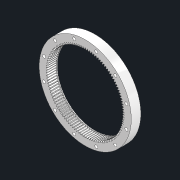
# Autodesk Inventor part: unit-ring_gear
Saved by Autodesk Inventor 2021 (Build 250183000, 183)
## iProperties
Created: 2021-07-12
Part Number: unit-ring_gear
Material: ABS プラスチック
Document SubType Name: Modeling
Designer: yuta0
Density: 1.06 g/cm^3
Appearance: 滑らか - 白
Mass: 40.8022 g
Surface Area: 244.347 cm^2
Volume: 38.4926 cm^3
Author: yuta0
Autodesk Inventor part; units mm, degrees
ref_plane "YZ Plane" through (0, 0, 0) normal (1, 0, 0) x (0, 1, 0)
ref_plane "XZ Plane" through (0, 0, 0) normal (0, 1, 0) x (-1, 0, 0)
ref_plane "XY Plane" through (0, 0, 0) normal (0, 0, 1) x (1, 0, 0)
sketch "スケッチ1" plane through (0, 0, 0) normal (0, 0, 1) x (1, 0, 0)
  arc A0 (3.605, -57.0442) -> (4.2313, -54.7448) centre (-9.8704, -52.1391) ccw
  arc A1 (2.8046, -57.0892) -> (3.605, -57.0442) centre (0, 0) ccw
  arc A2 (1.9248, -54.8743) -> (2.8046, -57.0892) centre (15.6461, -50.7061) ccw
  arc A3 (1.155, -54.8959) -> (1.9248, -54.8743) centre (0, 0) ccw
  arc A4 (0.4008, -57.1566) -> (1.155, -54.8959) centre (-12.7783, -51.5036) ccw
  arc A5 (-0.4008, -57.1566) -> (0.4008, -57.1566) centre (0, 0) ccw
  arc A6 (-1.155, -54.8959) -> (-0.4008, -57.1566) centre (12.7783, -51.5036) ccw
  arc A7 (-1.9248, -54.8743) -> (-1.155, -54.8959) centre (0, 0) ccw
  arc A8 (-2.8046, -57.0892) -> (-1.9248, -54.8743) centre (-15.6461, -50.7061) ccw
  arc A9 (-3.605, -57.0442) -> (-2.8046, -57.0892) centre (0, 0) ccw
  arc A10 (-4.2313, -54.7448) -> (-3.605, -57.0442) centre (9.8704, -52.1391) ccw
  arc A11 (-4.9986, -54.68) -> (-4.2313, -54.7448) centre (0, 0) ccw
  arc A12 (-6.0012, -56.8421) -> (-4.9986, -54.68) centre (-18.4646, -49.7491) ccw
  arc A13 (-6.7978, -56.7524) -> (-6.0012, -56.8421) centre (0, 0) ccw
  arc A14 (-7.2942, -54.4214) -> (-6.7978, -56.7524) centre (6.9314, -52.6105) ccw
  arc A15 (-8.0567, -54.3137) -> (-7.2942, -54.4214) centre (0, 0) ccw
  arc A16 (-9.1789, -56.4162) -> (-8.0567, -54.3137) centre (-21.225, -48.6355) ccw
  arc A17 (-9.9692, -56.2819) -> (-9.1789, -56.4162) centre (0, 0) ccw
  arc A18 (-10.3341, -53.9268) -> (-9.9692, -56.2819) centre (3.9706, -52.9164) ccw
  arc A19 (-11.0894, -53.7765) -> (-10.3341, -53.9268) centre (0, 0) ccw
  arc A20 (-12.3278, -55.8128) -> (-11.0894, -53.7765) centre (-23.9186, -47.3689) ccw
  arc A21 (-13.1093, -55.6344) -> (-12.3278, -55.8128) centre (0, 0) ccw
  arc A22 (-13.3416, -53.2625) -> (-13.1093, -55.6344) centre (0.9973, -53.0558) ccw
  arc A23 (-14.0872, -53.0702) -> (-13.3416, -53.2625) centre (0, 0) ccw
  arc A24 (-15.4378, -55.0337) -> (-14.0872, -53.0702) centre (-26.537, -45.9533) ccw
  arc A25 (-16.2081, -54.8118) -> (-15.4378, -55.0337) centre (0, 0) ccw
  arc A26 (-16.307, -52.4306) -> (-16.2081, -54.8118) centre (-1.9791, -53.0282) ccw
  arc A27 (-17.0407, -52.1968) -> (-16.307, -52.4306) centre (0, 0) ccw
  arc A28 (-18.4993, -54.0816) -> (-17.0407, -52.1968) centre (-29.0718, -44.393) ccw
  arc A29 (-19.256, -53.8168) -> (-18.4993, -54.0816) centre (0, 0) ccw
  arc A30 (-19.2212, -51.4338) -> (-19.256, -53.8168) centre (-4.9493, -52.8339) ccw
  arc A31 (-19.9406, -51.1592) -> (-19.2212, -51.4338) centre (0, 0) ccw
  arc A32 (-21.5026, -52.9592) -> (-19.9406, -51.1592) centre (-31.5152, -42.6931) ccw
  arc A33 (-22.2432, -52.6524) -> (-21.5026, -52.9592) centre (0, 0) ccw
  arc A34 (-22.0749, -50.2752) -> (-22.2432, -52.6524) centre (-7.904, -52.4732) ccw
  arc A35 (-22.7778, -49.9606) -> (-22.0749, -50.2752) centre (0, 0) ccw
  arc A36 (-24.4382, -51.6702) -> (-22.7778, -49.9606) centre (-33.8595, -40.8589) ccw
  arc A37 (-25.1605, -51.3224) -> (-24.4382, -51.6702) centre (0, 0) ccw
  arc A38 (-24.8591, -48.9583) -> (-25.1605, -51.3224) centre (-10.8337, -51.9475) ccw
  arc A39 (-25.5433, -48.6049) -> (-24.8591, -48.9583) centre (0, 0) ccw
  arc A40 (-27.2969, -50.2187) -> (-25.5433, -48.6049) centre (-36.0972, -38.8961) ccw
  arc A41 (-27.9985, -49.8309) -> (-27.2969, -50.2187) centre (0, 0) ccw
  arc A42 (-27.5651, -47.4874) -> (-27.9985, -49.8309) centre (-13.7294, -51.2583) ccw
  arc A43 (-28.2284, -47.0962) -> (-27.5651, -47.4874) centre (0, 0) ccw
  arc A44 (-30.0698, -48.6091) -> (-28.2284, -47.0962) centre (-38.2213, -36.8109) ccw
  arc A45 (-30.7485, -48.1826) -> (-30.0698, -48.6091) centre (0, 0) ccw
  arc A46 (-30.1844, -45.8671) -> (-30.7485, -48.1826) centre (-16.5819, -50.4079) ccw
  arc A47 (-30.8247, -45.4393) -> (-30.1844, -45.8671) centre (0, 0) ccw
  arc A48 (-32.748, -46.8466) -> (-30.8247, -45.4393) centre (-40.2252, -34.6099) ccw
  arc A49 (-33.4018, -46.3828) -> (-32.748, -46.8466) centre (0, 0) ccw
  arc A50 (-32.7087, -44.1025) -> (-33.4018, -46.3828) centre (-19.3822, -49.3988) ccw
  arc A51 (-33.324, -43.6395) -> (-32.7087, -44.1025) centre (0, 0) ccw
  arc A52 (-35.3232, -44.9368) -> (-33.324, -43.6395) centre (-42.1025, -32.3) ccw
  arc A53 (-35.9499, -44.4369) -> (-35.3232, -44.9368) centre (0, 0) ccw
  arc A54 (-35.1301, -42.1992) -> (-35.9499, -44.4369) centre (-22.1215, -48.2343) ccw
  arc A55 (-35.7184, -41.7023) -> (-35.1301, -42.1992) centre (0, 0) ccw
  arc A56 (-37.7873, -42.8855) -> (-35.7184, -41.7023) centre (-43.8473, -29.8885) ccw
  arc A57 (-38.385, -42.3513) -> (-37.7873, -42.8855) centre (0, 0) ccw
  arc A58 (-37.4409, -40.163) -> (-38.385, -42.3513) centre (-24.7912, -46.9181) ccw
  arc A59 (-38.0005, -39.634) -> (-37.4409, -40.163) centre (0, 0) ccw
  arc A60 (-40.1324, -40.6993) -> (-38.0005, -39.634) centre (-45.4542, -27.3829) ccw
  arc A61 (-40.6993, -40.1324) -> (-40.1324, -40.6993) centre (0, 0) ccw
  arc A62 (-39.634, -38.0005) -> (-40.6993, -40.1324) centre (-27.3829, -45.4542) ccw
  arc A63 (-40.163, -37.4409) -> (-39.634, -38.0005) centre (0, 0) ccw
  arc A64 (-42.3513, -38.385) -> (-40.163, -37.4409) centre (-46.9181, -24.7912) ccw
  arc A65 (-42.8855, -37.7873) -> (-42.3513, -38.385) centre (0, 0) ccw
  arc A66 (-41.7023, -35.7184) -> (-42.8855, -37.7873) centre (-29.8885, -43.8473) ccw
  arc A67 (-42.1992, -35.1301) -> (-41.7023, -35.7184) centre (0, 0) ccw
  arc A68 (-44.4369, -35.9499) -> (-42.1992, -35.1301) centre (-48.2343, -22.1215) ccw
  arc A69 (-44.9368, -35.3232) -> (-44.4369, -35.9499) centre (0, 0) ccw
  arc A70 (-43.6395, -33.324) -> (-44.9368, -35.3232) centre (-32.3, -42.1025) ccw
  arc A71 (-44.1025, -32.7087) -> (-43.6395, -33.324) centre (0, 0) ccw
  arc A72 (-46.3828, -33.4018) -> (-44.1025, -32.7087) centre (-49.3988, -19.3822) ccw
  arc A73 (-46.8466, -32.748) -> (-46.3828, -33.4018) centre (0, 0) ccw
  arc A74 (-45.4393, -30.8247) -> (-46.8466, -32.748) centre (-34.6099, -40.2252) ccw
  arc A75 (-45.8671, -30.1844) -> (-45.4393, -30.8247) centre (0, 0) ccw
  arc A76 (-48.1826, -30.7485) -> (-45.8671, -30.1844) centre (-50.4079, -16.5819) ccw
  arc A77 (-48.6091, -30.0698) -> (-48.1826, -30.7485) centre (0, 0) ccw
  arc A78 (-47.0962, -28.2284) -> (-48.6091, -30.0698) centre (-36.8109, -38.2213) ccw
  arc A79 (-47.4874, -27.5651) -> (-47.0962, -28.2284) centre (0, 0) ccw
  arc A80 (-49.8309, -27.9985) -> (-47.4874, -27.5651) centre (-51.2583, -13.7294) ccw
  arc A81 (-50.2187, -27.2969) -> (-49.8309, -27.9985) centre (0, 0) ccw
  arc A82 (-48.6049, -25.5433) -> (-50.2187, -27.2969) centre (-38.8961, -36.0972) ccw
  arc A83 (-48.9583, -24.8591) -> (-48.6049, -25.5433) centre (0, 0) ccw
  arc A84 (-51.3224, -25.1605) -> (-48.9583, -24.8591) centre (-51.9475, -10.8337) ccw
  arc A85 (-51.6702, -24.4382) -> (-51.3224, -25.1605) centre (0, 0) ccw
  arc A86 (-49.9606, -22.7778) -> (-51.6702, -24.4382) centre (-40.8589, -33.8595) ccw
  arc A87 (-50.2752, -22.0749) -> (-49.9606, -22.7778) centre (0, 0) ccw
  arc A88 (-52.6524, -22.2432) -> (-50.2752, -22.0749) centre (-52.4732, -7.904) ccw
  arc A89 (-52.9592, -21.5026) -> (-52.6524, -22.2432) centre (0, 0) ccw
  arc A90 (-51.1592, -19.9406) -> (-52.9592, -21.5026) centre (-42.6931, -31.5152) ccw
  arc A91 (-51.4338, -19.2212) -> (-51.1592, -19.9406) centre (0, 0) ccw
  arc A92 (-53.8168, -19.256) -> (-51.4338, -19.2212) centre (-52.8339, -4.9493) ccw
  arc A93 (-54.0816, -18.4993) -> (-53.8168, -19.256) centre (0, 0) ccw
  arc A94 (-52.1968, -17.0407) -> (-54.0816, -18.4993) centre (-44.393, -29.0718) ccw
  arc A95 (-52.4306, -16.307) -> (-52.1968, -17.0407) centre (0, 0) ccw
  arc A96 (-54.8118, -16.2081) -> (-52.4306, -16.307) centre (-53.0282, -1.9791) ccw
  arc A97 (-55.0337, -15.4378) -> (-54.8118, -16.2081) centre (0, 0) ccw
  arc A98 (-53.0702, -14.0872) -> (-55.0337, -15.4378) centre (-45.9533, -26.537) ccw
  arc A99 (-53.2625, -13.3416) -> (-53.0702, -14.0872) centre (0, 0) ccw
  arc A100 (-55.6344, -13.1093) -> (-53.2625, -13.3416) centre (-53.0558, 0.9973) ccw
  arc A101 (-55.8128, -12.3278) -> (-55.6344, -13.1093) centre (0, 0) ccw
  arc A102 (-53.7765, -11.0894) -> (-55.8128, -12.3278) centre (-47.3689, -23.9186) ccw
  arc A103 (-53.9268, -10.3341) -> (-53.7765, -11.0894) centre (0, 0) ccw
  arc A104 (-56.2819, -9.9692) -> (-53.9268, -10.3341) centre (-52.9164, 3.9706) ccw
  arc A105 (-56.4162, -9.1789) -> (-56.2819, -9.9692) centre (0, 0) ccw
  arc A106 (-54.3137, -8.0567) -> (-56.4162, -9.1789) centre (-48.6355, -21.225) ccw
  arc A107 (-54.4214, -7.2942) -> (-54.3137, -8.0567) centre (0, 0) ccw
  arc A108 (-56.7524, -6.7978) -> (-54.4214, -7.2942) centre (-52.6105, 6.9314) ccw
  arc A109 (-56.8421, -6.0012) -> (-56.7524, -6.7978) centre (0, 0) ccw
  arc A110 (-54.68, -4.9986) -> (-56.8421, -6.0012) centre (-49.7491, -18.4646) ccw
  arc A111 (-54.7448, -4.2313) -> (-54.68, -4.9986) centre (0, 0) ccw
  arc A112 (-57.0442, -3.605) -> (-54.7448, -4.2313) centre (-52.1391, 9.8704) ccw
  arc A113 (-57.0892, -2.8046) -> (-57.0442, -3.605) centre (0, 0) ccw
  arc A114 (-54.8743, -1.9248) -> (-57.0892, -2.8046) centre (-50.7061, -15.6461) ccw
  arc A115 (-54.8959, -1.155) -> (-54.8743, -1.9248) centre (0, 0) ccw
  arc A116 (-57.1566, -0.4008) -> (-54.8959, -1.155) centre (-51.5036, 12.7783) ccw
  arc A117 (-57.1566, 0.4008) -> (-57.1566, -0.4008) centre (0, 0) ccw
  arc A118 (-54.8959, 1.155) -> (-57.1566, 0.4008) centre (-51.5036, -12.7783) ccw
  arc A119 (-54.8743, 1.9248) -> (-54.8959, 1.155) centre (0, 0) ccw
  arc A120 (-57.0892, 2.8046) -> (-54.8743, 1.9248) centre (-50.7061, 15.6461) ccw
  arc A121 (-57.0442, 3.605) -> (-57.0892, 2.8046) centre (0, 0) ccw
  arc A122 (-54.7448, 4.2313) -> (-57.0442, 3.605) centre (-52.1391, -9.8704) ccw
  arc A123 (-54.68, 4.9986) -> (-54.7448, 4.2313) centre (0, 0) ccw
  arc A124 (-56.8421, 6.0012) -> (-54.68, 4.9986) centre (-49.7491, 18.4646) ccw
  arc A125 (-56.7524, 6.7978) -> (-56.8421, 6.0012) centre (0, 0) ccw
  arc A126 (-54.4214, 7.2942) -> (-56.7524, 6.7978) centre (-52.6105, -6.9314) ccw
  arc A127 (-54.3137, 8.0567) -> (-54.4214, 7.2942) centre (0, 0) ccw
  arc A128 (-56.4162, 9.1789) -> (-54.3137, 8.0567) centre (-48.6355, 21.225) ccw
  arc A129 (-56.2819, 9.9692) -> (-56.4162, 9.1789) centre (0, 0) ccw
  arc A130 (-53.9268, 10.3341) -> (-56.2819, 9.9692) centre (-52.9164, -3.9706) ccw
  arc A131 (-53.7765, 11.0894) -> (-53.9268, 10.3341) centre (0, 0) ccw
  arc A132 (-55.8128, 12.3278) -> (-53.7765, 11.0894) centre (-47.3689, 23.9186) ccw
  arc A133 (-55.6344, 13.1093) -> (-55.8128, 12.3278) centre (0, 0) ccw
  arc A134 (-53.2625, 13.3416) -> (-55.6344, 13.1093) centre (-53.0558, -0.9973) ccw
  arc A135 (-53.0702, 14.0872) -> (-53.2625, 13.3416) centre (0, 0) ccw
  arc A136 (-55.0337, 15.4378) -> (-53.0702, 14.0872) centre (-45.9533, 26.537) ccw
  arc A137 (-54.8118, 16.2081) -> (-55.0337, 15.4378) centre (0, 0) ccw
  arc A138 (-52.4306, 16.307) -> (-54.8118, 16.2081) centre (-53.0282, 1.9791) ccw
  arc A139 (-52.1968, 17.0407) -> (-52.4306, 16.307) centre (0, 0) ccw
  arc A140 (-54.0816, 18.4993) -> (-52.1968, 17.0407) centre (-44.393, 29.0718) ccw
  arc A141 (-53.8168, 19.256) -> (-54.0816, 18.4993) centre (0, 0) ccw
  arc A142 (-51.4338, 19.2212) -> (-53.8168, 19.256) centre (-52.8339, 4.9493) ccw
  arc A143 (-51.1592, 19.9406) -> (-51.4338, 19.2212) centre (0, 0) ccw
  arc A144 (-52.9592, 21.5026) -> (-51.1592, 19.9406) centre (-42.6931, 31.5152) ccw
  arc A145 (-52.6524, 22.2432) -> (-52.9592, 21.5026) centre (0, 0) ccw
  arc A146 (-50.2752, 22.0749) -> (-52.6524, 22.2432) centre (-52.4732, 7.904) ccw
  arc A147 (-49.9606, 22.7778) -> (-50.2752, 22.0749) centre (0, 0) ccw
  arc A148 (-51.6702, 24.4382) -> (-49.9606, 22.7778) centre (-40.8589, 33.8595) ccw
  arc A149 (-51.3224, 25.1605) -> (-51.6702, 24.4382) centre (0, 0) ccw
  arc A150 (-48.9583, 24.8591) -> (-51.3224, 25.1605) centre (-51.9475, 10.8337) ccw
  arc A151 (-48.6049, 25.5433) -> (-48.9583, 24.8591) centre (0, 0) ccw
  arc A152 (-50.2187, 27.2969) -> (-48.6049, 25.5433) centre (-38.8961, 36.0972) ccw
  arc A153 (-49.8309, 27.9985) -> (-50.2187, 27.2969) centre (0, 0) ccw
  arc A154 (-47.4874, 27.5651) -> (-49.8309, 27.9985) centre (-51.2583, 13.7294) ccw
  arc A155 (-47.0962, 28.2284) -> (-47.4874, 27.5651) centre (0, 0) ccw
  arc A156 (-48.6091, 30.0698) -> (-47.0962, 28.2284) centre (-36.8109, 38.2213) ccw
  arc A157 (-48.1826, 30.7485) -> (-48.6091, 30.0698) centre (0, 0) ccw
  arc A158 (-45.8671, 30.1844) -> (-48.1826, 30.7485) centre (-50.4079, 16.5819) ccw
  arc A159 (-45.4393, 30.8247) -> (-45.8671, 30.1844) centre (0, 0) ccw
  arc A160 (-46.8466, 32.748) -> (-45.4393, 30.8247) centre (-34.6099, 40.2252) ccw
  arc A161 (-46.3828, 33.4018) -> (-46.8466, 32.748) centre (0, 0) ccw
  arc A162 (-44.1025, 32.7087) -> (-46.3828, 33.4018) centre (-49.3988, 19.3822) ccw
  arc A163 (-43.6395, 33.324) -> (-44.1025, 32.7087) centre (0, 0) ccw
  arc A164 (-44.9368, 35.3232) -> (-43.6395, 33.324) centre (-32.3, 42.1025) ccw
  arc A165 (-44.4369, 35.9499) -> (-44.9368, 35.3232) centre (0, 0) ccw
  arc A166 (-42.1992, 35.1301) -> (-44.4369, 35.9499) centre (-48.2343, 22.1215) ccw
  arc A167 (-41.7023, 35.7184) -> (-42.1992, 35.1301) centre (0, 0) ccw
  arc A168 (-42.8855, 37.7873) -> (-41.7023, 35.7184) centre (-29.8885, 43.8473) ccw
  arc A169 (-42.3513, 38.385) -> (-42.8855, 37.7873) centre (0, 0) ccw
  arc A170 (-40.163, 37.4409) -> (-42.3513, 38.385) centre (-46.9181, 24.7912) ccw
  arc A171 (-39.634, 38.0005) -> (-40.163, 37.4409) centre (0, 0) ccw
  arc A172 (-40.6993, 40.1324) -> (-39.634, 38.0005) centre (-27.3829, 45.4542) ccw
  arc A173 (-40.1324, 40.6993) -> (-40.6993, 40.1324) centre (0, 0) ccw
  arc A174 (-38.0005, 39.634) -> (-40.1324, 40.6993) centre (-45.4542, 27.3829) ccw
  arc A175 (-37.4409, 40.163) -> (-38.0005, 39.634) centre (0, 0) ccw
  arc A176 (-38.385, 42.3513) -> (-37.4409, 40.163) centre (-24.7912, 46.9181) ccw
  arc A177 (-37.7873, 42.8855) -> (-38.385, 42.3513) centre (0, 0) ccw
  arc A178 (-35.7184, 41.7023) -> (-37.7873, 42.8855) centre (-43.8473, 29.8885) ccw
  arc A179 (-35.1301, 42.1992) -> (-35.7184, 41.7023) centre (0, 0) ccw
  arc A180 (-35.9499, 44.4369) -> (-35.1301, 42.1992) centre (-22.1215, 48.2343) ccw
  arc A181 (-35.3232, 44.9368) -> (-35.9499, 44.4369) centre (0, 0) ccw
  arc A182 (-33.324, 43.6395) -> (-35.3232, 44.9368) centre (-42.1025, 32.3) ccw
  arc A183 (-32.7087, 44.1025) -> (-33.324, 43.6395) centre (0, 0) ccw
  arc A184 (-33.4018, 46.3828) -> (-32.7087, 44.1025) centre (-19.3822, 49.3988) ccw
  arc A185 (-32.748, 46.8466) -> (-33.4018, 46.3828) centre (0, 0) ccw
  arc A186 (-30.8247, 45.4393) -> (-32.748, 46.8466) centre (-40.2252, 34.6099) ccw
  arc A187 (-30.1844, 45.8671) -> (-30.8247, 45.4393) centre (0, 0) ccw
  arc A188 (-30.7485, 48.1826) -> (-30.1844, 45.8671) centre (-16.5819, 50.4079) ccw
  arc A189 (-30.0698, 48.6091) -> (-30.7485, 48.1826) centre (0, 0) ccw
  arc A190 (-28.2284, 47.0962) -> (-30.0698, 48.6091) centre (-38.2213, 36.8109) ccw
  arc A191 (-27.5651, 47.4874) -> (-28.2284, 47.0962) centre (0, 0) ccw
  arc A192 (-27.9985, 49.8309) -> (-27.5651, 47.4874) centre (-13.7294, 51.2583) ccw
  arc A193 (-27.2969, 50.2187) -> (-27.9985, 49.8309) centre (0, 0) ccw
  arc A194 (-25.5433, 48.6049) -> (-27.2969, 50.2187) centre (-36.0972, 38.8961) ccw
  arc A195 (-24.8591, 48.9583) -> (-25.5433, 48.6049) centre (0, 0) ccw
  arc A196 (-25.1605, 51.3224) -> (-24.8591, 48.9583) centre (-10.8337, 51.9475) ccw
  arc A197 (-24.4382, 51.6702) -> (-25.1605, 51.3224) centre (0, 0) ccw
  arc A198 (-22.7778, 49.9606) -> (-24.4382, 51.6702) centre (-33.8595, 40.8589) ccw
  arc A199 (-22.0749, 50.2752) -> (-22.7778, 49.9606) centre (0, 0) ccw
  arc A200 (-22.2432, 52.6524) -> (-22.0749, 50.2752) centre (-7.904, 52.4732) ccw
  arc A201 (-21.5026, 52.9592) -> (-22.2432, 52.6524) centre (0, 0) ccw
  arc A202 (-19.9406, 51.1592) -> (-21.5026, 52.9592) centre (-31.5152, 42.6931) ccw
  arc A203 (-19.2212, 51.4338) -> (-19.9406, 51.1592) centre (0, 0) ccw
  arc A204 (-19.256, 53.8168) -> (-19.2212, 51.4338) centre (-4.9493, 52.8339) ccw
  arc A205 (-18.4993, 54.0816) -> (-19.256, 53.8168) centre (0, 0) ccw
  arc A206 (-17.0407, 52.1968) -> (-18.4993, 54.0816) centre (-29.0718, 44.393) ccw
  arc A207 (-16.307, 52.4306) -> (-17.0407, 52.1968) centre (0, 0) ccw
  arc A208 (-16.2081, 54.8118) -> (-16.307, 52.4306) centre (-1.9791, 53.0282) ccw
  arc A209 (-15.4378, 55.0337) -> (-16.2081, 54.8118) centre (0, 0) ccw
  arc A210 (-14.0872, 53.0702) -> (-15.4378, 55.0337) centre (-26.537, 45.9533) ccw
  arc A211 (-13.3416, 53.2625) -> (-14.0872, 53.0702) centre (0, 0) ccw
  arc A212 (-13.1093, 55.6344) -> (-13.3416, 53.2625) centre (0.9973, 53.0558) ccw
  arc A213 (-12.3278, 55.8128) -> (-13.1093, 55.6344) centre (0, 0) ccw
  arc A214 (-11.0894, 53.7765) -> (-12.3278, 55.8128) centre (-23.9186, 47.3689) ccw
  arc A215 (-10.3341, 53.9268) -> (-11.0894, 53.7765) centre (0, 0) ccw
  arc A216 (-9.9692, 56.2819) -> (-10.3341, 53.9268) centre (3.9706, 52.9164) ccw
  arc A217 (-9.1789, 56.4162) -> (-9.9692, 56.2819) centre (0, 0) ccw
  arc A218 (-8.0567, 54.3137) -> (-9.1789, 56.4162) centre (-21.225, 48.6355) ccw
  arc A219 (-7.2942, 54.4214) -> (-8.0567, 54.3137) centre (0, 0) ccw
  arc A220 (-6.7978, 56.7524) -> (-7.2942, 54.4214) centre (6.9314, 52.6105) ccw
  arc A221 (-6.0012, 56.8421) -> (-6.7978, 56.7524) centre (0, 0) ccw
  arc A222 (-4.9986, 54.68) -> (-6.0012, 56.8421) centre (-18.4646, 49.7491) ccw
  arc A223 (-4.2313, 54.7448) -> (-4.9986, 54.68) centre (0, 0) ccw
  arc A224 (-3.605, 57.0442) -> (-4.2313, 54.7448) centre (9.8704, 52.1391) ccw
  arc A225 (-2.8046, 57.0892) -> (-3.605, 57.0442) centre (0, 0) ccw
  arc A226 (-1.9248, 54.8743) -> (-2.8046, 57.0892) centre (-15.6461, 50.7061) ccw
  arc A227 (-1.155, 54.8959) -> (-1.9248, 54.8743) centre (0, 0) ccw
  arc A228 (-0.4008, 57.1566) -> (-1.155, 54.8959) centre (12.7783, 51.5036) ccw
  arc A229 (0.4008, 57.1566) -> (-0.4008, 57.1566) centre (0, 0) ccw
  arc A230 (1.155, 54.8959) -> (0.4008, 57.1566) centre (-12.7783, 51.5036) ccw
  arc A231 (1.9248, 54.8743) -> (1.155, 54.8959) centre (0, 0) ccw
  arc A232 (2.8046, 57.0892) -> (1.9248, 54.8743) centre (15.6461, 50.7061) ccw
  arc A233 (3.605, 57.0442) -> (2.8046, 57.0892) centre (0, 0) ccw
  arc A234 (4.2313, 54.7448) -> (3.605, 57.0442) centre (-9.8704, 52.1391) ccw
  arc A235 (4.9986, 54.68) -> (4.2313, 54.7448) centre (0, 0) ccw
  arc A236 (6.0012, 56.8421) -> (4.9986, 54.68) centre (18.4646, 49.7491) ccw
  arc A237 (6.7978, 56.7524) -> (6.0012, 56.8421) centre (0, 0) ccw
  arc A238 (7.2942, 54.4214) -> (6.7978, 56.7524) centre (-6.9314, 52.6105) ccw
  arc A239 (8.0567, 54.3137) -> (7.2942, 54.4214) centre (0, 0) ccw
  arc A240 (9.1789, 56.4162) -> (8.0567, 54.3137) centre (21.225, 48.6355) ccw
  arc A241 (9.9692, 56.2819) -> (9.1789, 56.4162) centre (0, 0) ccw
  arc A242 (10.3341, 53.9268) -> (9.9692, 56.2819) centre (-3.9706, 52.9164) ccw
  arc A243 (11.0894, 53.7765) -> (10.3341, 53.9268) centre (0, 0) ccw
  arc A244 (12.3278, 55.8128) -> (11.0894, 53.7765) centre (23.9186, 47.3689) ccw
  arc A245 (13.1093, 55.6344) -> (12.3278, 55.8128) centre (0, 0) ccw
  arc A246 (13.3416, 53.2625) -> (13.1093, 55.6344) centre (-0.9973, 53.0558) ccw
  arc A247 (14.0872, 53.0702) -> (13.3416, 53.2625) centre (0, 0) ccw
  arc A248 (15.4378, 55.0337) -> (14.0872, 53.0702) centre (26.537, 45.9533) ccw
  arc A249 (16.2081, 54.8118) -> (15.4378, 55.0337) centre (0, 0) ccw
  arc A250 (16.307, 52.4306) -> (16.2081, 54.8118) centre (1.9791, 53.0282) ccw
  arc A251 (17.0407, 52.1968) -> (16.307, 52.4306) centre (0, 0) ccw
  arc A252 (18.4993, 54.0816) -> (17.0407, 52.1968) centre (29.0718, 44.393) ccw
  arc A253 (19.256, 53.8168) -> (18.4993, 54.0816) centre (0, 0) ccw
  arc A254 (19.2212, 51.4338) -> (19.256, 53.8168) centre (4.9493, 52.8339) ccw
  arc A255 (19.9406, 51.1592) -> (19.2212, 51.4338) centre (0, 0) ccw
  arc A256 (21.5026, 52.9592) -> (19.9406, 51.1592) centre (31.5152, 42.6931) ccw
  arc A257 (22.2432, 52.6524) -> (21.5026, 52.9592) centre (0, 0) ccw
  arc A258 (22.0749, 50.2752) -> (22.2432, 52.6524) centre (7.904, 52.4732) ccw
  arc A259 (22.7778, 49.9606) -> (22.0749, 50.2752) centre (0, 0) ccw
  arc A260 (24.4382, 51.6702) -> (22.7778, 49.9606) centre (33.8595, 40.8589) ccw
  arc A261 (25.1605, 51.3224) -> (24.4382, 51.6702) centre (0, 0) ccw
  arc A262 (24.8591, 48.9583) -> (25.1605, 51.3224) centre (10.8337, 51.9475) ccw
  arc A263 (25.5433, 48.6049) -> (24.8591, 48.9583) centre (0, 0) ccw
  arc A264 (27.2969, 50.2187) -> (25.5433, 48.6049) centre (36.0972, 38.8961) ccw
  arc A265 (27.9985, 49.8309) -> (27.2969, 50.2187) centre (0, 0) ccw
  arc A266 (27.5651, 47.4874) -> (27.9985, 49.8309) centre (13.7294, 51.2583) ccw
  arc A267 (28.2284, 47.0962) -> (27.5651, 47.4874) centre (0, 0) ccw
  arc A268 (30.0698, 48.6091) -> (28.2284, 47.0962) centre (38.2213, 36.8109) ccw
  arc A269 (30.7485, 48.1826) -> (30.0698, 48.6091) centre (0, 0) ccw
  arc A270 (30.1844, 45.8671) -> (30.7485, 48.1826) centre (16.5819, 50.4079) ccw
  arc A271 (30.8247, 45.4393) -> (30.1844, 45.8671) centre (0, 0) ccw
  arc A272 (32.748, 46.8466) -> (30.8247, 45.4393) centre (40.2252, 34.6099) ccw
  arc A273 (33.4018, 46.3828) -> (32.748, 46.8466) centre (0, 0) ccw
  arc A274 (32.7087, 44.1025) -> (33.4018, 46.3828) centre (19.3822, 49.3988) ccw
  arc A275 (33.324, 43.6395) -> (32.7087, 44.1025) centre (0, 0) ccw
  arc A276 (35.3232, 44.9368) -> (33.324, 43.6395) centre (42.1025, 32.3) ccw
  arc A277 (35.9499, 44.4369) -> (35.3232, 44.9368) centre (0, 0) ccw
  arc A278 (35.1301, 42.1992) -> (35.9499, 44.4369) centre (22.1215, 48.2343) ccw
  arc A279 (35.7184, 41.7023) -> (35.1301, 42.1992) centre (0, 0) ccw
  arc A280 (37.7873, 42.8855) -> (35.7184, 41.7023) centre (43.8473, 29.8885) ccw
  arc A281 (38.385, 42.3513) -> (37.7873, 42.8855) centre (0, 0) ccw
  arc A282 (37.4409, 40.163) -> (38.385, 42.3513) centre (24.7912, 46.9181) ccw
  arc A283 (38.0005, 39.634) -> (37.4409, 40.163) centre (0, 0) ccw
  arc A284 (40.1324, 40.6993) -> (38.0005, 39.634) centre (45.4542, 27.3829) ccw
  arc A285 (40.6993, 40.1324) -> (40.1324, 40.6993) centre (0, 0) ccw
  arc A286 (39.634, 38.0005) -> (40.6993, 40.1324) centre (27.3829, 45.4542) ccw
  arc A287 (40.163, 37.4409) -> (39.634, 38.0005) centre (0, 0) ccw
  arc A288 (42.3513, 38.385) -> (40.163, 37.4409) centre (46.9181, 24.7912) ccw
  arc A289 (42.8855, 37.7873) -> (42.3513, 38.385) centre (0, 0) ccw
  arc A290 (41.7023, 35.7184) -> (42.8855, 37.7873) centre (29.8885, 43.8473) ccw
  arc A291 (42.1992, 35.1301) -> (41.7023, 35.7184) centre (0, 0) ccw
  arc A292 (44.4369, 35.9499) -> (42.1992, 35.1301) centre (48.2343, 22.1215) ccw
  arc A293 (44.9368, 35.3232) -> (44.4369, 35.9499) centre (0, 0) ccw
  arc A294 (43.6395, 33.324) -> (44.9368, 35.3232) centre (32.3, 42.1025) ccw
  arc A295 (44.1025, 32.7087) -> (43.6395, 33.324) centre (0, 0) ccw
  arc A296 (46.3828, 33.4018) -> (44.1025, 32.7087) centre (49.3988, 19.3822) ccw
  arc A297 (46.8466, 32.748) -> (46.3828, 33.4018) centre (0, 0) ccw
  arc A298 (45.4393, 30.8247) -> (46.8466, 32.748) centre (34.6099, 40.2252) ccw
  arc A299 (45.8671, 30.1844) -> (45.4393, 30.8247) centre (0, 0) ccw
  arc A300 (48.1826, 30.7485) -> (45.8671, 30.1844) centre (50.4079, 16.5819) ccw
  arc A301 (48.6091, 30.0698) -> (48.1826, 30.7485) centre (0, 0) ccw
  arc A302 (47.0962, 28.2284) -> (48.6091, 30.0698) centre (36.8109, 38.2213) ccw
  arc A303 (47.4874, 27.5651) -> (47.0962, 28.2284) centre (0, 0) ccw
  arc A304 (49.8309, 27.9985) -> (47.4874, 27.5651) centre (51.2583, 13.7294) ccw
  arc A305 (50.2187, 27.2969) -> (49.8309, 27.9985) centre (0, 0) ccw
  arc A306 (48.6049, 25.5433) -> (50.2187, 27.2969) centre (38.8961, 36.0972) ccw
  arc A307 (48.9583, 24.8591) -> (48.6049, 25.5433) centre (0, 0) ccw
  arc A308 (51.3224, 25.1605) -> (48.9583, 24.8591) centre (51.9475, 10.8337) ccw
  arc A309 (51.6702, 24.4382) -> (51.3224, 25.1605) centre (0, 0) ccw
  arc A310 (49.9606, 22.7778) -> (51.6702, 24.4382) centre (40.8589, 33.8595) ccw
  arc A311 (50.2752, 22.0749) -> (49.9606, 22.7778) centre (0, 0) ccw
  arc A312 (52.6524, 22.2432) -> (50.2752, 22.0749) centre (52.4732, 7.904) ccw
  arc A313 (52.9592, 21.5026) -> (52.6524, 22.2432) centre (0, 0) ccw
  arc A314 (51.1592, 19.9406) -> (52.9592, 21.5026) centre (42.6931, 31.5152) ccw
  arc A315 (51.4338, 19.2212) -> (51.1592, 19.9406) centre (0, 0) ccw
  arc A316 (53.8168, 19.256) -> (51.4338, 19.2212) centre (52.8339, 4.9493) ccw
  arc A317 (54.0816, 18.4993) -> (53.8168, 19.256) centre (0, 0) ccw
  arc A318 (52.1968, 17.0407) -> (54.0816, 18.4993) centre (44.393, 29.0718) ccw
  arc A319 (52.4306, 16.307) -> (52.1968, 17.0407) centre (0, 0) ccw
  arc A320 (54.8118, 16.2081) -> (52.4306, 16.307) centre (53.0282, 1.9791) ccw
  arc A321 (55.0337, 15.4378) -> (54.8118, 16.2081) centre (0, 0) ccw
  arc A322 (53.0702, 14.0872) -> (55.0337, 15.4378) centre (45.9533, 26.537) ccw
  arc A323 (53.2625, 13.3416) -> (53.0702, 14.0872) centre (0, 0) ccw
  arc A324 (55.6344, 13.1093) -> (53.2625, 13.3416) centre (53.0558, -0.9973) ccw
  arc A325 (55.8128, 12.3278) -> (55.6344, 13.1093) centre (0, 0) ccw
  arc A326 (53.7765, 11.0894) -> (55.8128, 12.3278) centre (47.3689, 23.9186) ccw
  arc A327 (53.9268, 10.3341) -> (53.7765, 11.0894) centre (0, 0) ccw
  arc A328 (56.2819, 9.9692) -> (53.9268, 10.3341) centre (52.9164, -3.9706) ccw
  arc A329 (56.4162, 9.1789) -> (56.2819, 9.9692) centre (0, 0) ccw
  arc A330 (54.3137, 8.0567) -> (56.4162, 9.1789) centre (48.6355, 21.225) ccw
  arc A331 (54.4214, 7.2942) -> (54.3137, 8.0567) centre (0, 0) ccw
  arc A332 (56.7524, 6.7978) -> (54.4214, 7.2942) centre (52.6105, -6.9314) ccw
  arc A333 (56.8421, 6.0012) -> (56.7524, 6.7978) centre (0, 0) ccw
  arc A334 (54.68, 4.9986) -> (56.8421, 6.0012) centre (49.7491, 18.4646) ccw
  arc A335 (54.7448, 4.2313) -> (54.68, 4.9986) centre (0, 0) ccw
  arc A336 (57.0442, 3.605) -> (54.7448, 4.2313) centre (52.1391, -9.8704) ccw
  arc A337 (57.0892, 2.8046) -> (57.0442, 3.605) centre (0, 0) ccw
  arc A338 (54.8743, 1.9248) -> (57.0892, 2.8046) centre (50.7061, 15.6461) ccw
  arc A339 (54.8959, 1.155) -> (54.8743, 1.9248) centre (0, 0) ccw
  arc A340 (57.1566, 0.4008) -> (54.8959, 1.155) centre (51.5036, -12.7783) ccw
  arc A341 (57.1566, -0.4008) -> (57.1566, 0.4008) centre (0, 0) ccw
  arc A342 (54.8959, -1.155) -> (57.1566, -0.4008) centre (51.5036, 12.7783) ccw
  arc A343 (54.8743, -1.9248) -> (54.8959, -1.155) centre (0, 0) ccw
  arc A344 (57.0892, -2.8046) -> (54.8743, -1.9248) centre (50.7061, -15.6461) ccw
  arc A345 (57.0442, -3.605) -> (57.0892, -2.8046) centre (0, 0) ccw
  arc A346 (54.7448, -4.2313) -> (57.0442, -3.605) centre (52.1391, 9.8704) ccw
  arc A347 (54.68, -4.9986) -> (54.7448, -4.2313) centre (0, 0) ccw
  arc A348 (56.8421, -6.0012) -> (54.68, -4.9986) centre (49.7491, -18.4646) ccw
  arc A349 (56.7524, -6.7978) -> (56.8421, -6.0012) centre (0, 0) ccw
  arc A350 (54.4214, -7.2942) -> (56.7524, -6.7978) centre (52.6105, 6.9314) ccw
  arc A351 (54.3137, -8.0567) -> (54.4214, -7.2942) centre (0, 0) ccw
  arc A352 (56.4162, -9.1789) -> (54.3137, -8.0567) centre (48.6355, -21.225) ccw
  arc A353 (56.2819, -9.9692) -> (56.4162, -9.1789) centre (0, 0) ccw
  arc A354 (53.9268, -10.3341) -> (56.2819, -9.9692) centre (52.9164, 3.9706) ccw
  arc A355 (53.7765, -11.0894) -> (53.9268, -10.3341) centre (0, 0) ccw
  arc A356 (55.8128, -12.3278) -> (53.7765, -11.0894) centre (47.3689, -23.9186) ccw
  arc A357 (55.6344, -13.1093) -> (55.8128, -12.3278) centre (0, 0) ccw
  arc A358 (53.2625, -13.3416) -> (55.6344, -13.1093) centre (53.0558, 0.9973) ccw
  arc A359 (53.0702, -14.0872) -> (53.2625, -13.3416) centre (0, 0) ccw
  arc A360 (55.0337, -15.4378) -> (53.0702, -14.0872) centre (45.9533, -26.537) ccw
  arc A361 (54.8118, -16.2081) -> (55.0337, -15.4378) centre (0, 0) ccw
  arc A362 (52.4306, -16.307) -> (54.8118, -16.2081) centre (53.0282, -1.9791) ccw
  arc A363 (52.1968, -17.0407) -> (52.4306, -16.307) centre (0, 0) ccw
  arc A364 (54.0816, -18.4993) -> (52.1968, -17.0407) centre (44.393, -29.0718) ccw
  arc A365 (53.8168, -19.256) -> (54.0816, -18.4993) centre (0, 0) ccw
  arc A366 (51.4338, -19.2212) -> (53.8168, -19.256) centre (52.8339, -4.9493) ccw
  arc A367 (51.1592, -19.9406) -> (51.4338, -19.2212) centre (0, 0) ccw
  arc A368 (52.9592, -21.5026) -> (51.1592, -19.9406) centre (42.6931, -31.5152) ccw
  arc A369 (52.6524, -22.2432) -> (52.9592, -21.5026) centre (0, 0) ccw
  arc A370 (50.2752, -22.0749) -> (52.6524, -22.2432) centre (52.4732, -7.904) ccw
  arc A371 (49.9606, -22.7778) -> (50.2752, -22.0749) centre (0, 0) ccw
  arc A372 (51.6702, -24.4382) -> (49.9606, -22.7778) centre (40.8589, -33.8595) ccw
  arc A373 (51.3224, -25.1605) -> (51.6702, -24.4382) centre (0, 0) ccw
  arc A374 (48.9583, -24.8591) -> (51.3224, -25.1605) centre (51.9475, -10.8337) ccw
  arc A375 (48.6049, -25.5433) -> (48.9583, -24.8591) centre (0, 0) ccw
  arc A376 (50.2187, -27.2969) -> (48.6049, -25.5433) centre (38.8961, -36.0972) ccw
  arc A377 (49.8309, -27.9985) -> (50.2187, -27.2969) centre (0, 0) ccw
  arc A378 (47.4874, -27.5651) -> (49.8309, -27.9985) centre (51.2583, -13.7294) ccw
  arc A379 (47.0962, -28.2284) -> (47.4874, -27.5651) centre (0, 0) ccw
  arc A380 (48.6091, -30.0698) -> (47.0962, -28.2284) centre (36.8109, -38.2213) ccw
  arc A381 (48.1826, -30.7485) -> (48.6091, -30.0698) centre (0, 0) ccw
  arc A382 (45.8671, -30.1844) -> (48.1826, -30.7485) centre (50.4079, -16.5819) ccw
  arc A383 (45.4393, -30.8247) -> (45.8671, -30.1844) centre (0, 0) ccw
  arc A384 (46.8466, -32.748) -> (45.4393, -30.8247) centre (34.6099, -40.2252) ccw
  arc A385 (46.3828, -33.4018) -> (46.8466, -32.748) centre (0, 0) ccw
  arc A386 (44.1025, -32.7087) -> (46.3828, -33.4018) centre (49.3988, -19.3822) ccw
  arc A387 (43.6395, -33.324) -> (44.1025, -32.7087) centre (0, 0) ccw
  arc A388 (44.9368, -35.3232) -> (43.6395, -33.324) centre (32.3, -42.1025) ccw
  arc A389 (44.4369, -35.9499) -> (44.9368, -35.3232) centre (0, 0) ccw
  arc A390 (42.1992, -35.1301) -> (44.4369, -35.9499) centre (48.2343, -22.1215) ccw
  arc A391 (41.7023, -35.7184) -> (42.1992, -35.1301) centre (0, 0) ccw
  arc A392 (42.8855, -37.7873) -> (41.7023, -35.7184) centre (29.8885, -43.8473) ccw
  arc A393 (42.3513, -38.385) -> (42.8855, -37.7873) centre (0, 0) ccw
  arc A394 (40.163, -37.4409) -> (42.3513, -38.385) centre (46.9181, -24.7912) ccw
  arc A395 (39.634, -38.0005) -> (40.163, -37.4409) centre (0, 0) ccw
  arc A396 (40.6993, -40.1324) -> (39.634, -38.0005) centre (27.3829, -45.4542) ccw
  arc A397 (40.1324, -40.6993) -> (40.6993, -40.1324) centre (0, 0) ccw
  arc A398 (38.0005, -39.634) -> (40.1324, -40.6993) centre (45.4542, -27.3829) ccw
  arc A399 (37.4409, -40.163) -> (38.0005, -39.634) centre (0, 0) ccw
  arc A400 (38.385, -42.3513) -> (37.4409, -40.163) centre (24.7912, -46.9181) ccw
  arc A401 (37.7873, -42.8855) -> (38.385, -42.3513) centre (0, 0) ccw
  arc A402 (35.7184, -41.7023) -> (37.7873, -42.8855) centre (43.8473, -29.8885) ccw
  arc A403 (35.1301, -42.1992) -> (35.7184, -41.7023) centre (0, 0) ccw
  arc A404 (35.9499, -44.4369) -> (35.1301, -42.1992) centre (22.1215, -48.2343) ccw
  arc A405 (35.3232, -44.9368) -> (35.9499, -44.4369) centre (0, 0) ccw
  arc A406 (33.324, -43.6395) -> (35.3232, -44.9368) centre (42.1025, -32.3) ccw
  arc A407 (32.7087, -44.1025) -> (33.324, -43.6395) centre (0, 0) ccw
  arc A408 (33.4018, -46.3828) -> (32.7087, -44.1025) centre (19.3822, -49.3988) ccw
  arc A409 (32.748, -46.8466) -> (33.4018, -46.3828) centre (0, 0) ccw
  arc A410 (30.8247, -45.4393) -> (32.748, -46.8466) centre (40.2252, -34.6099) ccw
  arc A411 (30.1844, -45.8671) -> (30.8247, -45.4393) centre (0, 0) ccw
  arc A412 (30.7485, -48.1826) -> (30.1844, -45.8671) centre (16.5819, -50.4079) ccw
  arc A413 (30.0698, -48.6091) -> (30.7485, -48.1826) centre (0, 0) ccw
  arc A414 (28.2284, -47.0962) -> (30.0698, -48.6091) centre (38.2213, -36.8109) ccw
  arc A415 (27.5651, -47.4874) -> (28.2284, -47.0962) centre (0, 0) ccw
  arc A416 (27.9985, -49.8309) -> (27.5651, -47.4874) centre (13.7294, -51.2583) ccw
  arc A417 (27.2969, -50.2187) -> (27.9985, -49.8309) centre (0, 0) ccw
  arc A418 (25.5433, -48.6049) -> (27.2969, -50.2187) centre (36.0972, -38.8961) ccw
  arc A419 (24.8591, -48.9583) -> (25.5433, -48.6049) centre (0, 0) ccw
  arc A420 (25.1605, -51.3224) -> (24.8591, -48.9583) centre (10.8337, -51.9475) ccw
  arc A421 (24.4382, -51.6702) -> (25.1605, -51.3224) centre (0, 0) ccw
  arc A422 (22.7778, -49.9606) -> (24.4382, -51.6702) centre (33.8595, -40.8589) ccw
  arc A423 (22.0749, -50.2752) -> (22.7778, -49.9606) centre (0, 0) ccw
  arc A424 (22.2432, -52.6524) -> (22.0749, -50.2752) centre (7.904, -52.4732) ccw
  arc A425 (21.5026, -52.9592) -> (22.2432, -52.6524) centre (0, 0) ccw
  arc A426 (19.9406, -51.1592) -> (21.5026, -52.9592) centre (31.5152, -42.6931) ccw
  arc A427 (19.2212, -51.4338) -> (19.9406, -51.1592) centre (0, 0) ccw
  arc A428 (19.256, -53.8168) -> (19.2212, -51.4338) centre (4.9493, -52.8339) ccw
  arc A429 (18.4993, -54.0816) -> (19.256, -53.8168) centre (0, 0) ccw
  arc A430 (17.0407, -52.1968) -> (18.4993, -54.0816) centre (29.0718, -44.393) ccw
  arc A431 (16.307, -52.4306) -> (17.0407, -52.1968) centre (0, 0) ccw
  arc A432 (16.2081, -54.8118) -> (16.307, -52.4306) centre (1.9791, -53.0282) ccw
  arc A433 (15.4378, -55.0337) -> (16.2081, -54.8118) centre (0, 0) ccw
  arc A434 (14.0872, -53.0702) -> (15.4378, -55.0337) centre (26.537, -45.9533) ccw
  arc A435 (13.3416, -53.2625) -> (14.0872, -53.0702) centre (0, 0) ccw
  arc A436 (13.1093, -55.6344) -> (13.3416, -53.2625) centre (-0.9973, -53.0558) ccw
  arc A437 (12.3278, -55.8128) -> (13.1093, -55.6344) centre (0, 0) ccw
  arc A438 (11.0894, -53.7765) -> (12.3278, -55.8128) centre (23.9186, -47.3689) ccw
  arc A439 (10.3341, -53.9268) -> (11.0894, -53.7765) centre (0, 0) ccw
  arc A440 (9.9692, -56.2819) -> (10.3341, -53.9268) centre (-3.9706, -52.9164) ccw
  arc A441 (9.1789, -56.4162) -> (9.9692, -56.2819) centre (0, 0) ccw
  arc A442 (8.0567, -54.3137) -> (9.1789, -56.4162) centre (21.225, -48.6355) ccw
  arc A443 (7.2942, -54.4214) -> (8.0567, -54.3137) centre (0, 0) ccw
  arc A444 (6.7978, -56.7524) -> (7.2942, -54.4214) centre (-6.9314, -52.6105) ccw
  arc A445 (6.0012, -56.8421) -> (6.7978, -56.7524) centre (0, 0) ccw
  arc A446 (4.9986, -54.68) -> (6.0012, -56.8421) centre (18.4646, -49.7491) ccw
  arc A447 (4.2313, -54.7448) -> (4.9986, -54.68) centre (0, 0) ccw
  circle A448 centre (0, 0) radius 67.5
  dimension "d0" = 135
  constraints: 896 point on circle, 449 centre point, 1 coincident, 1346 other
  measures "d0" diameter of A448
extrude "押し出し1" add sketch "スケッチ1" along normal mid plane 13
sketch "スケッチ5" plane through (0, 0, -6.5) normal (0, 0, -1) x (-1, 0, 0)
  circle A0 centre (0, 0) radius 67.5 projected
  arc A1 (-48.9583, 24.8591) -> (-51.3224, 25.1605) centre (-51.9475, 10.8337) ccw projected
  circle A2 centre (0, 0) radius 54.908
  constraints: 1 coincident, 3 other
extrude "押し出し3" add sketch "スケッチ5" along normal blind 1
sketch "スケッチ2" plane through (0, 0, 6.5) normal (0, 0, 1) x (1, 0, 0)
  circle A0 centre (0, 0) radius 62.5
  point P0 (-16.1762, 60.3704)
  point P1 (-44.1942, 44.1942)
  point P2 (-60.3704, 16.1762)
  point P3 (-60.3704, -16.1762)
  point P4 (-44.1942, -44.1942)
  point P5 (-16.1762, -60.3704)
  point P6 (16.1762, -60.3704)
  point P7 (44.1942, -44.1942)
  point P8 (60.3704, -16.1762)
  point P9 (60.3704, 16.1762)
  point P10 (44.1942, 44.1942)
  point P11 (16.1762, 60.3704)
  dimension "d3" = 125
  dimension "d6" = 360
  dimension "d21" = 0
  constraints: 1 coincident, 16 other
  measures "d21" vertical distance of point (16.176, 60.37) point (-16.176, 60.37)
hole "穴1" at (-16.1762, 60.3704, 6.5) at (-44.1942, 44.1942, 6.5) at (-60.3704, 16.1762, 6.5) at (-60.3704, -16.1762, 6.5) at (-44.1942, -44.1942, 6.5) at (-16.1762, -60.3704, 6.5) at (16.1762, -60.3704, 6.5) at (44.1942, -44.1942, 6.5) at (60.3704, -16.1762, 6.5) at (60.3704, 16.1762, 6.5) at (44.1942, 44.1942, 6.5) at (16.1762, 60.3704, 6.5) direction (0, 0, -1) diameter 4.5 end through all clearance for "Flat Head Machine Screw" size "M4" standard "Ansi Metric M Profile"
sketch "スケッチ3" plane through (0, 0, 6.5) normal (0, 0, 1) x (1, 0, 0)
  circle A0 centre (-16.1762, 60.3704) radius 2.25 projected
  circle A1 centre (-44.1942, 44.1942) radius 2.25 projected
  circle A2 centre (0, 0) radius 67.5 projected
  circle A3 centre (-44.1942, 44.1942) radius 5
  circle A4 centre (-16.1762, 60.3704) radius 5
  circle A5 centre (0, 0) radius 62.5
  point P0 (-40.52, 47.5855)
  point P1 (-20.9502, 58.8841)
  point P2 (-17.4703, 65.2)
  point P3 (-47.7297, 47.7297)
  constraints: 2 centre point, 2 tangent, 3 other
